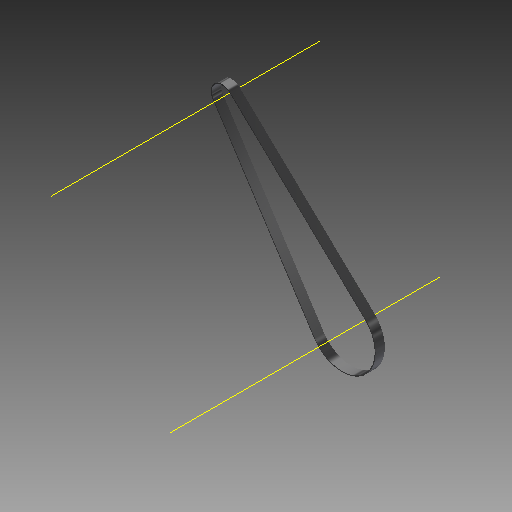
# Autodesk Inventor part: Synchronous Belt
Saved by Autodesk Inventor 2019.4 (Build 234330000, 330)
## iProperties
Created: 2020-01-23
Part Number: Synchronous Belt
Material: Rubber
Document SubType Name: Modeling
Designer: admin
Density: 0.93 g/cm^3
Appearance: Rubber - Black - Version 1.1
Mass: 8.184 g
Surface Area: 187 cm^2
Volume: 8.8 cm^3
CustomPartVersion: 1
Author: admin
Autodesk Inventor part; units mm, degrees
sketch "Sketch Path" plane through (0, 0, 0) normal (0, 0, 1) x (1, 0, 0)
  arc A0 (-95.1813, -9.9018) -> (-40.4421, 35.5127) centre (-65.1307, 9.5739) ccw
  arc A1 (-186.9011, 174.9123) -> (-205.1475, 159.7742) centre (-195.1307, 166.2661) ccw
  line L0 (-186.9011, 174.9123) -> (-40.4421, 35.5127)
  line L1 (-95.1813, -9.9018) -> (-205.1475, 159.7742)
  constraints: 4 end point, 4 point on circle, 2 centre point
ref_plane "Cross Section Plane" through (-40.4421, 35.5127, 0) normal (-0.7243, 0.6894, 0) x (0, 0, 1)
ref_plane "Work Plane2" through (-65.1307, 9.5739, 0) normal (-1, 0, 0) x (0, 0, 1)
ref_plane "Work Plane3" through (-195.1307, 166.2661, 0) normal (0.1846, -0.9828, 0) x (0, 0, 1)
sketch "Cross Section" plane through (-40.4421, 35.5127, 0) normal (-0.7243, 0.6894, 0) x (0, 0, 1)
  line L0 (-5, 0.5) -> (5, 0.5)
  line L1 (5, 0.5) -> (5, -0.5)
  line L2 (5, -0.5) -> (-5, -0.5)
  line L3 (-5, -0.5) -> (-5, 0.5)
  line L4 (-5, 0) -> (5, 0) construction
  point P0 (0, 0)
  point P1 (0, 0)
  dimension "d0" = 10
  dimension "d4" = 0.5
  dimension "d5" = 0.5
  constraints: 10 end point, 3 midpoint, 2 parallel, 1 coincident, 1 horizontal, 1 perpendicular, 1 other
  measures "d0" distance between parallel lines of L1 L3
  measures "d4" distance between parallel lines of L2 L4
  measures "d5" distance between parallel lines of L4 L0
sweep "Belt" add profiles "Cross Section" path "Sketch Path"
equation "\"d0\" = da_B"
equation "\"d4\" = da_a"
equation "\"d5\" = da_a2"
equation "\"da_B\" = 10"
equation "\"da_pb\" = 5"
equation "\"da_a\" = 0.5"
equation "\"da_S\" = 2.65"
equation "\"da_Beta\" = 20deg"
equation "\"da_Ht\" = 1.2"
equation "\"da_H\" = 2.2"
equation "\"da_a2\" = 0.5"
body "Solid1"
